Autodesk Fusion 360 part; units mm, degrees
note: some values were not read from the file. Chosen so that the rebuilt part matches the saved one: which bodies a step acts on; which pieces of a blend or face edit are solid. Set by a fixed rule: which sketch regions a step uses.
(part 3 of 4)
  spline S7 degree 5 poles (-3.4009, 1.0262) (-3.3954, 1.0308) (-3.3845, 1.0401) (-3.3681, 1.0541) (-3.3463, 1.0727) (-3.3193, 1.0962) (-3.2925, 1.1198) (-3.2658, 1.1434) (-3.2393, 1.1672) (-3.213, 1.191) (-3.1868, 1.215) (-3.1608, 1.239) (-3.135, 1.2632) (-3.1094, 1.2874) (-3.084, 1.3118) (-3.0587, 1.3362) (-3.0337, 1.3607) (-3.0088, 1.3854) (-2.9841, 1.4101) (-2.9595, 1.4349) (-2.9352, 1.4598) (-2.9111, 1.4848) (-2.8871, 1.5099) (-2.8634, 1.5352) (-2.8398, 1.5604) (-2.8165, 1.5858) (-2.7933, 1.6113) (-2.7703, 1.6369) (-2.7476, 1.6626) (-2.725, 1.6883) (-2.7027, 1.7142) (-2.6805, 1.7401) (-2.6586, 1.7662) (-2.6369, 1.7923) (-2.6154, 1.8185) (-2.5941, 1.8448) (-2.5731, 1.8713) (-2.5522, 1.8977) (-2.5316, 1.9243) (-2.5112, 1.951) (-2.491, 1.9778) (-2.4711, 2.0047) (-2.4514, 2.0316) (-2.432, 2.0587) (-2.4128, 2.0858) (-2.3939, 2.113) (-2.3751, 2.1403) (-2.3567, 2.1678) (-2.3385, 2.1953) (-2.3205, 2.2228) (-2.3029, 2.2505) (-2.2855, 2.2783) (-2.2684, 2.3062) (-2.2516, 2.3342) (-2.2352, 2.3622) (-2.219, 2.3904) (-2.203, 2.4187) (-2.1874, 2.447) (-2.172, 2.4754) (-2.157, 2.5039) (-2.1423, 2.5326) (-2.1281, 2.5613) (-2.1144, 2.5902) (-2.1011, 2.6192) (-2.0883, 2.6484) (-2.0758, 2.6776) (-2.0636, 2.7069) (-2.0515, 2.7362) (-2.0398, 2.7656) (-2.0288, 2.7952) (-2.0187, 2.825) (-2.0118, 2.8491) (-2.0073, 2.8674) (-2.0047, 2.8797) (-2.0035, 2.8858) knots -1 -1 -1 -1 -1 -1 -0.98571429 -0.97142857 -0.95714286 -0.94285714 -0.92857143 -0.91428571 -0.9 -0.88571429 -0.87142857 -0.85714286 -0.84285714 -0.82857143 -0.81428571 -0.8 -0.78571429 -0.77142857 -0.75714286 -0.74285714 -0.72857143 -0.71428571 -0.7 -0.68571429 -0.67142857 -0.65714286 -0.64285714 -0.62857143 -0.61428571 -0.6 -0.58571429 -0.57142857 -0.55714286 -0.54285714 -0.52857143 -0.51428571 -0.5 -0.48571429 -0.47142857 -0.45714286 -0.44285714 -0.42857143 -0.41428571 -0.4 -0.38571429 -0.37142857 -0.35714286 -0.34285714 -0.32857143 -0.31428571 -0.3 -0.28571429 -0.27142857 -0.25714286 -0.24285714 -0.22857143 -0.21428571 -0.2 -0.18571429 -0.17142857 -0.15714286 -0.14285714 -0.12857143 -0.11428571 -0.1 -0.08571429 -0.07142857 -0.05714286 -0.04285714 -0.02857143 -0.01428571 0 0 0 0 0 0
  line L7 (-2.0035, 2.8858) -> (-1.9517, 3.1488)
  arc A15 (-1.0746, 3.7888) -> (-1.9517, 3.1488) centre (-1.1668, 2.9941) ccw
  arc A16 (-1.0746, 3.7888) -> (-0.8753, 3.7678) centre (0, 13.0546) ccw
  arc A17 (-0.1505, 2.9594) -> (-0.8753, 3.7678) centre (-0.9504, 2.9714) ccw
  line L8 (-0.1505, 2.9594) -> (-0.1545, 2.6915)
  spline S8 degree 5 poles (-0.1545, 2.6915) (-0.1546, 2.6852) (-0.1546, 2.6727) (-0.154, 2.6538) (-0.1523, 2.6288) (-0.1486, 2.5976) (-0.1439, 2.5664) (-0.1386, 2.5352) (-0.133, 2.504) (-0.127, 2.4728) (-0.1209, 2.4416) (-0.1144, 2.4104) (-0.1075, 2.3793) (-0.1001, 2.3482) (-0.0922, 2.3171) (-0.0838, 2.286) (-0.075, 2.255) (-0.0659, 2.224) (-0.0564, 2.193) (-0.0467, 2.1621) (-0.0368, 2.1312) (-0.0265, 2.1003) (-0.0159, 2.0694) (-0.005, 2.0386) (0.0062, 2.0078) (0.0178, 1.9771) (0.0296, 1.9464) (0.0417, 1.9157) (0.054, 1.885) (0.0667, 1.8544) (0.0795, 1.8238) (0.0927, 1.7933) (0.1061, 1.7628) (0.1197, 1.7323) (0.1336, 1.7019) (0.1478, 1.6716) (0.1622, 1.6412) (0.1768, 1.6109) (0.1917, 1.5807) (0.2068, 1.5505) (0.2221, 1.5203) (0.2377, 1.4902) (0.2535, 1.4601) (0.2695, 1.4301) (0.2858, 1.4001) (0.3023, 1.3701) (0.319, 1.3403) (0.3359, 1.3104) (0.3531, 1.2806) (0.3704, 1.2509) (0.388, 1.2212) (0.4058, 1.1916) (0.4238, 1.162) (0.442, 1.1324) (0.4604, 1.1029) (0.479, 1.0735) (0.4978, 1.0441) (0.5168, 1.0148) (0.5361, 0.9855) (0.5555, 0.9563) (0.5751, 0.9272) (0.5949, 0.8981) (0.615, 0.869) (0.6352, 0.84) (0.6556, 0.8111) (0.6762, 0.7823) (0.697, 0.7534) (0.718, 0.7247) (0.7391, 0.696) (0.7605, 0.6674) (0.782, 0.6388) (0.7994, 0.616) (0.8126, 0.599) (0.8214, 0.5876) (0.8258, 0.5819) knots 0 0 0 0 0 0 0.01428571 0.02857143 0.04285714 0.05714286 0.07142857 0.08571429 0.1 0.11428571 0.12857143 0.14285714 0.15714286 0.17142857 0.18571429 0.2 0.21428571 0.22857143 0.24285714 0.25714286 0.27142857 0.28571429 0.3 0.31428571 0.32857143 0.34285714 0.35714286 0.37142857 0.38571429 0.4 0.41428571 0.42857143 0.44285714 0.45714286 0.47142857 0.48571429 0.5 0.51428571 0.52857143 0.54285714 0.55714286 0.57142857 0.58571429 0.6 0.61428571 0.62857143 0.64285714 0.65714286 0.67142857 0.68571429 0.7 0.71428571 0.72857143 0.74285714 0.75714286 0.77142857 0.78571429 0.8 0.81428571 0.82857143 0.84285714 0.85714286 0.87142857 0.88571429 0.9 0.91428571 0.92857143 0.94285714 0.95714286 0.97142857 0.98571429 1 1 1 1 1 1
  arc A18 (0.8258, 0.5819) -> (1.7855, 0.6828) centre (0, 13.0546) ccw
  spline S9 degree 5 poles (1.7855, 0.6828) (1.7886, 0.6893) (1.7949, 0.7022) (1.8042, 0.7216) (1.8164, 0.7476) (1.8316, 0.78) (1.8465, 0.8124) (1.8613, 0.8449) (1.8758, 0.8773) (1.8902, 0.9098) (1.9043, 0.9424) (1.9183, 0.9749) (1.932, 1.0075) (1.9455, 1.04) (1.9589, 1.0726) (1.972, 1.1052) (1.985, 1.1378) (1.9977, 1.1704) (2.0102, 1.2031) (2.0225, 1.2357) (2.0346, 1.2684) (2.0465, 1.3011) (2.0581, 1.3337) (2.0696, 1.3664) (2.0808, 1.3991) (2.0918, 1.4318) (2.1026, 1.4645) (2.1132, 1.4972) (2.1235, 1.5299) (2.1336, 1.5626) (2.1435, 1.5953) (2.1532, 1.628) (2.1627, 1.6608) (2.1719, 1.6935) (2.1808, 1.7262) (2.1896, 1.7589) (2.1981, 1.7915) (2.2063, 1.8242) (2.2144, 1.8569) (2.2221, 1.8896) (2.2297, 1.9222) (2.2369, 1.9549) (2.244, 1.9875) (2.2507, 2.0201) (2.2572, 2.0527) (2.2634, 2.0853) (2.2694, 2.1179) (2.2751, 2.1504) (2.2806, 2.1829) (2.2858, 2.2155) (2.2906, 2.2479) (2.2952, 2.2804) (2.2995, 2.3128) (2.3034, 2.3452) (2.3071, 2.3775) (2.3104, 2.4098) (2.3135, 2.4421) (2.3162, 2.4744) (2.3187, 2.5066) (2.3209, 2.5388) (2.3226, 2.5709) (2.3239, 2.6029) (2.3247, 2.6349) (2.325, 2.6668) (2.3248, 2.6987) (2.3244, 2.7304) (2.3236, 2.7622) (2.3227, 2.7939) (2.3214, 2.8255) (2.3195, 2.857) (2.3166, 2.8883) (2.3131, 2.9132) (2.3097, 2.9317) (2.3071, 2.944) (2.3057, 2.9501) knots -1 -1 -1 -1 -1 -1 -0.98571429 -0.97142857 -0.95714286 -0.94285714 -0.92857143 -0.91428571 -0.9 -0.88571429 -0.87142857 -0.85714286 -0.84285714 -0.82857143 -0.81428571 -0.8 -0.78571429 -0.77142857 -0.75714286 -0.74285714 -0.72857143 -0.71428571 -0.7 -0.68571429 -0.67142857 -0.65714286 -0.64285714 -0.62857143 -0.61428571 -0.6 -0.58571429 -0.57142857 -0.55714286 -0.54285714 -0.52857143 -0.51428571 -0.5 -0.48571429 -0.47142857 -0.45714286 -0.44285714 -0.42857143 -0.41428571 -0.4 -0.38571429 -0.37142857 -0.35714286 -0.34285714 -0.32857143 -0.31428571 -0.3 -0.28571429 -0.27142857 -0.25714286 -0.24285714 -0.22857143 -0.21428571 -0.2 -0.18571429 -0.17142857 -0.15714286 -0.14285714 -0.12857143 -0.11428571 -0.1 -0.08571429 -0.07142857 -0.05714286 -0.04285714 -0.02857143 -0.01428571 0 0 0 0 0 0
  line L9 (2.3057, 2.9501) -> (2.2461, 3.2113)
  arc A19 (2.787, 4.1528) -> (2.2461, 3.2113) centre (3.026, 3.3893) ccw
  arc A20 (2.787, 4.1528) -> (2.9776, 4.2147) centre (0, 13.0546) ccw
  arc A21 (3.9686, 3.771) -> (2.9776, 4.2147) centre (3.233, 3.4565) ccw
  line L10 (3.9686, 3.771) -> (4.0739, 3.5246)
  spline S10 degree 5 poles (4.0739, 3.5246) (4.0764, 3.5188) (4.0815, 3.5074) (4.0897, 3.4904) (4.1015, 3.4682) (4.1175, 3.4412) (4.1345, 3.4146) (4.152, 3.3882) (4.1699, 3.3621) (4.188, 3.336) (4.2063, 3.31) (4.2249, 3.2841) (4.2438, 3.2585) (4.2633, 3.2331) (4.2831, 3.2079) (4.3034, 3.1829) (4.3241, 3.1582) (4.345, 3.1336) (4.3662, 3.1091) (4.3877, 3.0848) (4.4094, 3.0606) (4.4313, 3.0366) (4.4536, 3.0127) (4.4761, 2.989) (4.4988, 2.9654) (4.5219, 2.942) (4.5452, 2.9188) (4.5687, 2.8956) (4.5924, 2.8727) (4.6164, 2.8498) (4.6406, 2.8271) (4.665, 2.8046) (4.6897, 2.7822) (4.7145, 2.7599) (4.7396, 2.7378) (4.7649, 2.7158) (4.7904, 2.6939) (4.8161, 2.6722) (4.842, 2.6506) (4.8681, 2.6292) (4.8944, 2.6078) (4.9208, 2.5867) (4.9475, 2.5656) (4.9744, 2.5447) (5.0014, 2.5239) (5.0287, 2.5033) (5.0561, 2.4828) (5.0837, 2.4624) (5.1115, 2.4421) (5.1394, 2.422) (5.1675, 2.4021) (5.1958, 2.3822) (5.2243, 2.3625) (5.2529, 2.3429) (5.2818, 2.3235) (5.3107, 2.3042) (5.3399, 2.285) (5.3692, 2.2659) (5.3987, 2.247) (5.4283, 2.2282) (5.4581, 2.2096) (5.488, 2.191) (5.5181, 2.1727) (5.5484, 2.1544) (5.5788, 2.1363) (5.6093, 2.1183) (5.6401, 2.1004) (5.6709, 2.0827) (5.7019, 2.0651) (5.7331, 2.0476) (5.7644, 2.0303) (5.7895, 2.0166) (5.8085, 2.0063) (5.8211, 1.9995) (5.8275, 1.9961) knots 0 0 0 0 0 0 0.01428571 0.02857143 0.04285714 0.05714286 0.07142857 0.08571429 0.1 0.11428571 0.12857143 0.14285714 0.15714286 0.17142857 0.18571429 0.2 0.21428571 0.22857143 0.24285714 0.25714286 0.27142857 0.28571429 0.3 0.31428571 0.32857143 0.34285714 0.35714286 0.37142857 0.38571429 0.4 0.41428571 0.42857143 0.44285714 0.45714286 0.47142857 0.48571429 0.5 0.51428571 0.52857143 0.54285714 0.55714286 0.57142857 0.58571429 0.6 0.61428571 0.62857143 0.64285714 0.65714286 0.67142857 0.68571429 0.7 0.71428571 0.72857143 0.74285714 0.75714286 0.77142857 0.78571429 0.8 0.81428571 0.82857143 0.84285714 0.85714286 0.87142857 0.88571429 0.9 0.91428571 0.92857143 0.94285714 0.95714286 0.97142857 0.98571429 1 1 1 1 1 1
  arc A22 (5.8275, 1.9961) -> (6.6632, 2.4786) centre (0, 13.0546) ccw
  spline S11 degree 5 poles (6.6632, 2.4786) (6.6634, 2.4858) (6.6639, 2.5002) (6.6645, 2.5217) (6.6651, 2.5504) (6.6658, 2.5861) (6.6662, 2.6218) (6.6665, 2.6575) (6.6666, 2.6931) (6.6665, 2.7286) (6.6662, 2.7641) (6.6657, 2.7995) (6.665, 2.8348) (6.6641, 2.8701) (6.6631, 2.9053) (6.6618, 2.9404) (6.6603, 2.9754) (6.6587, 3.0104) (6.6568, 3.0453) (6.6548, 3.0801) (6.6526, 3.1149) (6.6501, 3.1496) (6.6475, 3.1842) (6.6447, 3.2187) (6.6416, 3.2531) (6.6384, 3.2875) (6.6349, 3.3217) (6.6313, 3.3559) (6.6274, 3.39) (6.6234, 3.424) (6.6191, 3.4579) (6.6147, 3.4917) (6.61, 3.5254) (6.6051, 3.5591) (6.6, 3.5926) (6.5947, 3.626) (6.5891, 3.6593) (6.5834, 3.6926) (6.5774, 3.7257) (6.5713, 3.7587) (6.5649, 3.7916) (6.5582, 3.8243) (6.5514, 3.857) (6.5443, 3.8896) (6.5369, 3.922) (6.5294, 3.9543) (6.5216, 3.9865) (6.5136, 4.0185) (6.5053, 4.0505) (6.4968, 4.0822) (6.4881, 4.1139) (6.4791, 4.1454) (6.4698, 4.1768) (6.4602, 4.2079) (6.4504, 4.239) (6.4403, 4.2699) (6.4299, 4.3006) (6.4194, 4.3312) (6.4085, 4.3616) (6.3974, 4.3919) (6.3859, 4.4219) (6.3741, 4.4517) (6.3618, 4.4813) (6.3491, 4.5105) (6.336, 4.5396) (6.3226, 4.5684) (6.3091, 4.5971) (6.2953, 4.6257) (6.2813, 4.654) (6.2667, 4.682) (6.2513, 4.7095) (6.238, 4.7307) (6.2274, 4.7463) (6.22, 4.7564) (6.2162, 4.7615) knots -1 -1 -1 -1 -1 -1 -0.98571429 -0.97142857 -0.95714286 -0.94285714 -0.92857143 -0.91428571 -0.9 -0.88571429 -0.87142857 -0.85714286 -0.84285714 -0.82857143 -0.81428571 -0.8 -0.78571429 -0.77142857 -0.75714286 -0.74285714 -0.72857143 -0.71428571 -0.7 -0.68571429 -0.67142857 -0.65714286 -0.64285714 -0.62857143 -0.61428571 -0.6 -0.58571429 -0.57142857 -0.55714286 -0.54285714 -0.52857143 -0.51428571 -0.5 -0.48571429 -0.47142857 -0.45714286 -0.44285714 -0.42857143 -0.41428571 -0.4 -0.38571429 -0.37142857 -0.35714286 -0.34285714 -0.32857143 -0.31428571 -0.3 -0.28571429 -0.27142857 -0.25714286 -0.24285714 -0.22857143 -0.21428571 -0.2 -0.18571429 -0.17142857 -0.15714286 -0.14285714 -0.12857143 -0.11428571 -0.1 -0.08571429 -0.07142857 -0.05714286 -0.04285714 -0.02857143 -0.01428571 0 0 0 0 0 0
  line L11 (6.2162, 4.7615) -> (6.0555, 4.9759)
  arc A23 (6.1668, 6.0559) -> (6.0555, 4.9759) centre (6.6957, 5.4557) ccw
  arc A24 (6.1668, 6.0559) -> (6.3157, 6.1901) centre (0, 13.0546) ccw
  arc A25 (7.4015, 6.1878) -> (6.3157, 6.1901) centre (6.8574, 5.6013) ccw
  line L12 (7.4015, 6.1878) -> (7.5979, 6.0055)
  spline S12 degree 5 poles (7.5979, 6.0055) (7.6025, 6.0013) (7.6119, 5.9929) (7.6262, 5.9807) (7.646, 5.9652) (7.6717, 5.947) (7.698, 5.9296) (7.7247, 5.9127) (7.7517, 5.8961) (7.7788, 5.8796) (7.8061, 5.8633) (7.8336, 5.8472) (7.8614, 5.8315) (7.8895, 5.8162) (7.9179, 5.8013) (7.9465, 5.7867) (7.9755, 5.7725) (8.0046, 5.7586) (8.034, 5.7449) (8.0634, 5.7314) (8.0931, 5.7181) (8.1229, 5.7051) (8.1529, 5.6923) (8.1831, 5.6798) (8.2135, 5.6675) (8.2441, 5.6555) (8.2748, 5.6437) (8.3057, 5.6322) (8.3368, 5.6209) (8.368, 5.6098) (8.3993, 5.5989) (8.4308, 5.5882) (8.4624, 5.5777) (8.4942, 5.5675) (8.5261, 5.5575) (8.5581, 5.5477) (8.5903, 5.5381) (8.6226, 5.5287) (8.6551, 5.5195) (8.6876, 5.5105) (8.7203, 5.5017) (8.7531, 5.4931) (8.786, 5.4848) (8.8191, 5.4766) (8.8522, 5.4686) (8.8855, 5.4608) (8.9189, 5.4532) (8.9524, 5.4458) (8.986, 5.4387) (9.0197, 5.4317) (9.0536, 5.4248) (9.0875, 5.4182) (9.1215, 5.4118) (9.1556, 5.4056) (9.1899, 5.3995) (9.2242, 5.3936) (9.2586, 5.388) (9.2931, 5.3825) (9.3278, 5.3772) (9.3625, 5.3721) (9.3973, 5.3672) (9.4322, 5.3624) (9.4671, 5.3579) (9.5022, 5.3535) (9.5374, 5.3493) (9.5726, 5.3453) (9.6079, 5.3415) (9.6433, 5.3378) (9.6788, 5.3344) (9.7144, 5.3311) (9.75, 5.328) (9.7786, 5.3257) (9.8001, 5.324) (9.8144, 5.3229) (9.8216, 5.3224) knots 0 0 0 0 0 0 0.01428571 0.02857143 0.04285714 0.05714286 0.07142857 0.08571429 0.1 0.11428571 0.12857143 0.14285714 0.15714286 0.17142857 0.18571429 0.2 0.21428571 0.22857143 0.24285714 0.25714286 0.27142857 0.28571429 0.3 0.31428571 0.32857143 0.34285714 0.35714286 0.37142857 0.38571429 0.4 0.41428571 0.42857143 0.44285714 0.45714286 0.47142857 0.48571429 0.5 0.51428571 0.52857143 0.54285714 0.55714286 0.57142857 0.58571429 0.6 0.61428571 0.62857143 0.64285714 0.65714286 0.67142857 0.68571429 0.7 0.71428571 0.72857143 0.74285714 0.75714286 0.77142857 0.78571429 0.8 0.81428571 0.82857143 0.84285714 0.85714286 0.87142857 0.88571429 0.9 0.91428571 0.92857143 0.94285714 0.95714286 0.97142857 0.98571429 1 1 1 1 1 1
  arc A26 (9.8216, 5.3224) -> (10.3888, 6.1031) centre (0, 13.0546) ccw
  spline S13 degree 5 poles (10.3888, 6.1031) (10.3861, 6.1098) (10.3806, 6.1231) (10.3724, 6.143) (10.3614, 6.1694) (10.3474, 6.2024) (10.3333, 6.2352) (10.319, 6.2679) (10.3046, 6.3004) (10.2901, 6.3328) (10.2754, 6.3651) (10.2605, 6.3973) (10.2455, 6.4292) (10.2304, 6.4611) (10.2151, 6.4928) (10.1997, 6.5244) (10.1841, 6.5558) (10.1684, 6.5871) (10.1525, 6.6182) (10.1364, 6.6492) (10.1203, 6.6801) (10.1039, 6.7108) (10.0875, 6.7413) (10.0708, 6.7717) (10.054, 6.8019) (10.0371, 6.832) (10.02, 6.8619) (10.0028, 6.8916) (9.9854, 6.9212) (9.9679, 6.9506) (9.9502, 6.9798) (9.9324, 7.0089) (9.9144, 7.0378) (9.8962, 7.0665) (9.8779, 7.0951) (9.8595, 7.1235) (9.8409, 7.1516) (9.8221, 7.1797) (9.8032, 7.2075) (9.7841, 7.2351) (9.7649, 7.2626) (9.7455, 7.2898) (9.726, 7.3169) (9.7062, 7.3437) (9.6864, 7.3703) (9.6663, 7.3968) (9.6461, 7.423) (9.6258, 7.449) (9.6052, 7.4749) (9.5845, 7.5004) (9.5637, 7.5258) (9.5426, 7.5509) (9.5214, 7.5758) (9.5, 7.6004) (9.4783, 7.6247) (9.4566, 7.6488) (9.4346, 7.6727) (9.4125, 7.6964) (9.3902, 7.7198) (9.3678, 7.7429) (9.3451, 7.7657) (9.3221, 7.7881) (9.2989, 7.81) (9.2753, 7.8316) (9.2516, 7.8528) (9.2276, 7.8737) (9.2036, 7.8944) (9.1794, 7.9149) (9.1551, 7.9351) (9.1304, 7.9548) (9.1051, 7.9736) (9.0843, 7.9876) (9.0683, 7.9975) (9.0574, 8.0038) (9.0519, 8.0068) knots -1 -1 -1 -1 -1 -1 -0.98571429 -0.97142857 -0.95714286 -0.94285714 -0.92857143 -0.91428571 -0.9 -0.88571429 -0.87142857 -0.85714286 -0.84285714 -0.82857143 -0.81428571 -0.8 -0.78571429 -0.77142857 -0.75714286 -0.74285714 -0.72857143 -0.71428571 -0.7 -0.68571429 -0.67142857 -0.65714286 -0.64285714 -0.62857143 -0.61428571 -0.6 -0.58571429 -0.57142857 -0.55714286 -0.54285714 -0.52857143 -0.51428571 -0.5 -0.48571429 -0.47142857 -0.45714286 -0.44285714 -0.42857143 -0.41428571 -0.4 -0.38571429 -0.37142857 -0.35714286 -0.34285714 -0.32857143 -0.31428571 -0.3 -0.28571429 -0.27142857 -0.25714286 -0.24285714 -0.22857143 -0.21428571 -0.2 -0.18571429 -0.17142857 -0.15714286 -0.14285714 -0.12857143 -0.11428571 -0.1 -0.08571429 -0.07142857 -0.05714286 -0.04285714 -0.02857143 -0.01428571 0 0 0 0 0 0
  line L13 (9.0519, 8.0068) -> (8.8179, 8.1373)
  arc A27 (8.4802, 9.1693) -> (8.8179, 8.1373) centre (9.2075, 8.836) ccw
  arc A28 (8.4802, 9.1693) -> (8.5618, 9.3524) centre (0, 13.0546) ccw
  arc A29 (9.5546, 9.7919) -> (8.5618, 9.3524) centre (9.2961, 9.0348) ccw
  line L14 (9.5546, 9.7919) -> (9.8082, 9.7053)
  spline S14 degree 5 poles (9.8082, 9.7053) (9.8141, 9.7033) (9.8261, 9.6994) (9.8441, 9.6941) (9.8685, 9.6881) (9.8993, 9.6819) (9.9304, 9.6767) (9.9617, 9.6721) (9.9932, 9.6678) (10.0246, 9.6638) (10.0562, 9.66) (10.0879, 9.6566) (10.1196, 9.6535) (10.1515, 9.6509) (10.1835, 9.6489) (10.2156, 9.6472) (10.2479, 9.646) (10.2802, 9.6451) (10.3125, 9.6445) (10.345, 9.6442) (10.3774, 9.6441) (10.41, 9.6444) (10.4426, 9.6449) (10.4753, 9.6457) (10.508, 9.6469) (10.5409, 9.6484) (10.5737, 9.6501) (10.6066, 9.6521) (10.6396, 9.6544) (10.6726, 9.657) (10.7057, 9.6598) (10.7388, 9.6628) (10.7719, 9.6661) (10.8051, 9.6697) (10.8383, 9.6735) (10.8716, 9.6776) (10.9049, 9.6819) (10.9382, 9.6865) (10.9716, 9.6913) (11.005, 9.6963) (11.0384, 9.7016) (11.0719, 9.7071) (11.1054, 9.7128) (11.1389, 9.7188) (11.1724, 9.725) (11.206, 9.7314) (11.2396, 9.7381) (11.2732, 9.7449) (11.3068, 9.752) (11.3405, 9.7593) (11.3741, 9.7669) (11.4078, 9.7746) (11.4415, 9.7826) (11.4752, 9.7908) (11.509, 9.7992) (11.5427, 9.8078) (11.5765, 9.8166) (11.6102, 9.8256) (11.644, 9.8349) (11.6778, 9.8443) (11.7116, 9.854) (11.7454, 9.8639) (11.7792, 9.8739) (11.813, 9.8842) (11.8468, 9.8947) (11.8807, 9.9053) (11.9145, 9.9162) (11.9483, 9.9273) (11.9821, 9.9386) (12.0159, 9.95) (12.0498, 9.9617) (12.0768, 9.9712) (12.0971, 9.9784) (12.1106, 9.9832) (12.1174, 9.9857) knots 0 0 0 0 0 0 0.01428571 0.02857143 0.04285714 0.05714286 0.07142857 0.08571429 0.1 0.11428571 0.12857143 0.14285714 0.15714286 0.17142857 0.18571429 0.2 0.21428571 0.22857143 0.24285714 0.25714286 0.27142857 0.28571429 0.3 0.31428571 0.32857143 0.34285714 0.35714286 0.37142857 0.38571429 0.4 0.41428571 0.42857143 0.44285714 0.45714286 0.47142857 0.48571429 0.5 0.51428571 0.52857143 0.54285714 0.55714286 0.57142857 0.58571429 0.6 0.61428571 0.62857143 0.64285714 0.65714286 0.67142857 0.68571429 0.7 0.71428571 0.72857143 0.74285714 0.75714286 0.77142857 0.78571429 0.8 0.81428571 0.82857143 0.84285714 0.85714286 0.87142857 0.88571429 0.9 0.91428571 0.92857143 0.94285714 0.95714286 0.97142857 0.98571429 1 1 1 1 1 1
  arc A30 (12.1174, 9.9857) -> (12.3181, 10.9296) centre (0, 13.0546) ccw
  spline S15 degree 5 poles (12.3181, 10.9296) (12.3129, 10.9346) (12.3025, 10.9445) (12.2869, 10.9594) (12.266, 10.979) (12.2399, 11.0035) (12.2136, 11.0277) (12.1873, 11.0518) (12.1609, 11.0756) (12.1344, 11.0993) (12.1079, 11.1228) (12.0813, 11.1461) (12.0545, 11.1693) (12.0278, 11.1922) (12.0009, 11.215) (11.9739, 11.2375) (11.9469, 11.2599) (11.9198, 11.2821) (11.8926, 11.3041) (11.8654, 11.3259) (11.8381, 11.3475) (11.8107, 11.3689) (11.7832, 11.39) (11.7557, 11.411) (11.728, 11.4318) (11.7003, 11.4524) (11.6726, 11.4728) (11.6447, 11.4929) (11.6168, 11.5129) (11.5889, 11.5326) (11.5608, 11.5521) (11.5327, 11.5714) (11.5045, 11.5905) (11.4762, 11.6094) (11.4479, 11.628) (11.4195, 11.6464) (11.3911, 11.6646) (11.3625, 11.6826) (11.3339, 11.7003) (11.3053, 11.7178) (11.2765, 11.7351) (11.2477, 11.7521) (11.2189, 11.7688) (11.1899, 11.7853) (11.1609, 11.8016) (11.1319, 11.8176) (11.1027, 11.8333) (11.0736, 11.8488) (11.0443, 11.8641) (11.015, 11.879) (10.9856, 11.8937) (10.9562, 11.9081) (10.9267, 11.9221) (10.8971, 11.9359) (10.8674, 11.9494) (10.8377, 11.9625) (10.808, 11.9754) (10.7782, 11.988) (10.7483, 12.0003) (10.7184, 12.0123) (10.6883, 12.0239) (10.6583, 12.035) (10.6281, 12.0457) (10.5978, 12.0558) (10.5675, 12.0655) (10.5371, 12.0749) (10.5067, 12.084) (10.4763, 12.0929) (10.4458, 12.1014) (10.4153, 12.1093) (10.3846, 12.1162) (10.3599, 12.1206) (10.3412, 12.1231) (10.3287, 12.1244) (10.3225, 12.125) knots -1 -1 -1 -1 -1 -1 -0.98571429 -0.97142857 -0.95714286 -0.94285714 -0.92857143 -0.91428571 -0.9 -0.88571429 -0.87142857 -0.85714286 -0.84285714 -0.82857143 -0.81428571 -0.8 -0.78571429 -0.77142857 -0.75714286 -0.74285714 -0.72857143 -0.71428571 -0.7 -0.68571429 -0.67142857 -0.65714286 -0.64285714 -0.62857143 -0.61428571 -0.6 -0.58571429 -0.57142857 -0.55714286 -0.54285714 -0.52857143 -0.51428571 -0.5 -0.48571429 -0.47142857 -0.45714286 -0.44285714 -0.42857143 -0.41428571 -0.4 -0.38571429 -0.37142857 -0.35714286 -0.34285714 -0.32857143 -0.31428571 -0.3 -0.28571429 -0.27142857 -0.25714286 -0.24285714 -0.22857143 -0.21428571 -0.2 -0.18571429 -0.17142857 -0.15714286 -0.14285714 -0.12857143 -0.11428571 -0.1 -0.08571429 -0.07142857 -0.05714286 -0.04285714 -0.02857143 -0.01428571 0 0 0 0 0 0
  line L15 (10.3225, 12.125) -> (10.0556, 12.149)
  arc A31 (9.3274, 12.9544) -> (10.0556, 12.149) centre (10.1274, 12.9458) ccw
  arc A32 (9.3274, 12.9544) -> (9.3274, 13.1548) centre (0, 13.0546) ccw
  arc A33 (10.0556, 13.9602) -> (9.3274, 13.1548) centre (10.1274, 13.1634) ccw
  line L16 (10.0556, 13.9602) -> (10.3225, 13.9842)
  spline S16 degree 5 poles (10.3225, 13.9842) (10.3287, 13.9848) (10.3412, 13.9861) (10.3599, 13.9886) (10.3846, 13.993) (10.4153, 13.9999) (10.4458, 14.0078) (10.4763, 14.0163) (10.5067, 14.0252) (10.5371, 14.0344) (10.5675, 14.0437) (10.5978, 14.0534) (10.6281, 14.0636) (10.6583, 14.0742) (10.6883, 14.0853) (10.7184, 14.0969) (10.7483, 14.1089) (10.7782, 14.1212) (10.808, 14.1338) (10.8377, 14.1467) (10.8674, 14.1599) (10.8971, 14.1733) (10.9267, 14.1871) (10.9562, 14.2011) (10.9856, 14.2155) (11.015, 14.2302) (11.0443, 14.2452) (11.0736, 14.2604) (11.1027, 14.2759) (11.1319, 14.2916) (11.1609, 14.3076) (11.1899, 14.3239) (11.2189, 14.3404) (11.2477, 14.3572) (11.2765, 14.3742) (11.3053, 14.3914) (11.3339, 14.4089) (11.3625, 14.4266) (11.3911, 14.4446) (11.4195, 14.4628) (11.4479, 14.4812) (11.4762, 14.4998) (11.5045, 14.5187) (11.5327, 14.5378) (11.5608, 14.5571) (11.5889, 14.5766) (11.6168, 14.5963) (11.6447, 14.6163) (11.6726, 14.6365) (11.7003, 14.6568) (11.728, 14.6774) (11.7557, 14.6982) (11.7832, 14.7192) (11.8107, 14.7404) (11.8381, 14.7618) (11.8654, 14.7833) (11.8926, 14.8051) (11.9198, 14.8271) (11.9469, 14.8493) (11.9739, 14.8717) (12.0009, 14.8942) (12.0278, 14.917) (12.0545, 14.9399) (12.0813, 14.9631) (12.1079, 14.9864) (12.1344, 15.0099) (12.1609, 15.0336) (12.1873, 15.0575) (12.2136, 15.0815) (12.2399, 15.1058) (12.266, 15.1302) (12.2869, 15.1499) (12.3025, 15.1647) (12.3129, 15.1746) (12.3181, 15.1796) knots 0 0 0 0 0 0 0.01428571 0.02857143 0.04285714 0.05714286 0.07142857 0.08571429 0.1 0.11428571 0.12857143 0.14285714 0.15714286 0.17142857 0.18571429 0.2 0.21428571 0.22857143 0.24285714 0.25714286 0.27142857 0.28571429 0.3 0.31428571 0.32857143 0.34285714 0.35714286 0.37142857 0.38571429 0.4 0.41428571 0.42857143 0.44285714 0.45714286 0.47142857 0.48571429 0.5 0.51428571 0.52857143 0.54285714 0.55714286 0.57142857 0.58571429 0.6 0.61428571 0.62857143 0.64285714 0.65714286 0.67142857 0.68571429 0.7 0.71428571 0.72857143 0.74285714 0.75714286 0.77142857 0.78571429 0.8 0.81428571 0.82857143 0.84285714 0.85714286 0.87142857 0.88571429 0.9 0.91428571 0.92857143 0.94285714 0.95714286 0.97142857 0.98571429 1 1 1 1 1 1
  arc A34 (12.3181, 15.1796) -> (12.1174, 16.1235) centre (0, 13.0546) ccw
  spline S17 degree 5 poles (12.1174, 16.1235) (12.1106, 16.126) (12.0971, 16.1308) (12.0768, 16.138) (12.0498, 16.1475) (12.0159, 16.1592) (11.9821, 16.1707) (11.9483, 16.1819) (11.9145, 16.193) (11.8807, 16.2039) (11.8468, 16.2146) (11.813, 16.225) (11.7792, 16.2353) (11.7454, 16.2454) (11.7116, 16.2552) (11.6778, 16.2649) (11.644, 16.2743) (11.6102, 16.2836) (11.5765, 16.2926) (11.5427, 16.3014) (11.509, 16.31) (11.4752, 16.3184) (11.4415, 16.3266) (11.4078, 16.3346) (11.3741, 16.3423) (11.3405, 16.3499) (11.3068, 16.3572) (11.2732, 16.3643) (11.2396, 16.3712) (11.206, 16.3778) (11.1724, 16.3842) (11.1389, 16.3904) (11.1054, 16.3964) (11.0719, 16.4021) (11.0384, 16.4076) (11.005, 16.4129) (10.9716, 16.418) (10.9382, 16.4228) (10.9049, 16.4273) (10.8716, 16.4316) (10.8383, 16.4357) (10.8051, 16.4395) (10.7719, 16.4431) (10.7388, 16.4464) (10.7057, 16.4495) (10.6726, 16.4523) (10.6396, 16.4548) (10.6066, 16.4571) (10.5737, 16.4591) (10.5409, 16.4608) (10.508, 16.4623) (10.4753, 16.4635) (10.4426, 16.4643) (10.41, 16.4649) (10.3774, 16.4651) (10.345, 16.465) (10.3125, 16.4647) (10.2802, 16.4641) (10.2479, 16.4632) (10.2156, 16.462) (10.1835, 16.4604) (10.1515, 16.4583) (10.1196, 16.4557) (10.0879, 16.4527) (10.0562, 16.4492) (10.0246, 16.4454) (9.9932, 16.4414) (9.9617, 16.4371) (9.9304, 16.4325) (9.8993, 16.4274) (9.8685, 16.4212) (9.8441, 16.4151) (9.8261, 16.4098) (9.8141, 16.4059) (9.8082, 16.4039) knots -1 -1 -1 -1 -1 -1 -0.98571429 -0.97142857 -0.95714286 -0.94285714 -0.92857143 -0.91428571 -0.9 -0.88571429 -0.87142857 -0.85714286 -0.84285714 -0.82857143 -0.81428571 -0.8 -0.78571429 -0.77142857 -0.75714286 -0.74285714 -0.72857143 -0.71428571 -0.7 -0.68571429 -0.67142857 -0.65714286 -0.64285714 -0.62857143 -0.61428571 -0.6 -0.58571429 -0.57142857 -0.55714286 -0.54285714 -0.52857143 -0.51428571 -0.5 -0.48571429 -0.47142857 -0.45714286 -0.44285714 -0.42857143 -0.41428571 -0.4 -0.38571429 -0.37142857 -0.35714286 -0.34285714 -0.32857143 -0.31428571 -0.3 -0.28571429 -0.27142857 -0.25714286 -0.24285714 -0.22857143 -0.21428571 -0.2 -0.18571429 -0.17142857 -0.15714286 -0.14285714 -0.12857143 -0.11428571 -0.1 -0.08571429 -0.07142857 -0.05714286 -0.04285714 -0.02857143 -0.01428571 0 0 0 0 0 0
  line L17 (9.8082, 16.4039) -> (9.5546, 16.3173)
  arc A35 (8.5618, 16.7569) -> (9.5546, 16.3173) centre (9.2961, 17.0744) ccw
  arc A36 (8.5618, 16.7569) -> (8.4802, 16.94) centre (0, 13.0546) ccw
  arc A37 (8.8179, 17.9719) -> (8.4802, 16.94) centre (9.2075, 17.2732) ccw
  line L18 (8.8179, 17.9719) -> (9.0519, 18.1024)
  spline S18 degree 5 poles (9.0519, 18.1024) (9.0574, 18.1055) (9.0683, 18.1117) (9.0843, 18.1216) (9.1051, 18.1357) (9.1304, 18.1544) (9.1551, 18.1741) (9.1794, 18.1943) (9.2036, 18.2148) (9.2276, 18.2355) (9.2516, 18.2564) (9.2753, 18.2776) (9.2989, 18.2992) (9.3221, 18.3211) (9.3451, 18.3435) (9.3678, 18.3663) (9.3902, 18.3895) (9.4125, 18.4129) (9.4346, 18.4365) (9.4566, 18.4604) (9.4783, 18.4845) (9.5, 18.5088) (9.5214, 18.5334) (9.5426, 18.5583) (9.5637, 18.5834) (9.5845, 18.6088) (9.6052, 18.6344) (9.6258, 18.6602) (9.6461, 18.6862) (9.6663, 18.7124) (9.6864, 18.7389) (9.7062, 18.7655) (9.726, 18.7924) (9.7455, 18.8194) (9.7649, 18.8467) (9.7841, 18.8741) (9.8032, 18.9017) (9.8221, 18.9296) (9.8409, 18.9576) (9.8595, 18.9858) (9.8779, 19.0141) (9.8962, 19.0427) (9.9144, 19.0714) (9.9324, 19.1003) (9.9502, 19.1294) (9.9679, 19.1586) (9.9854, 19.188) (10.0028, 19.2176) (10.02, 19.2474) (10.0371, 19.2773) (10.054, 19.3073) (10.0708, 19.3375) (10.0875, 19.3679) (10.1039, 19.3985) (10.1203, 19.4291) (10.1364, 19.46) (10.1525, 19.491) (10.1684, 19.5221) (10.1841, 19.5534) (10.1997, 19.5848) (10.2151, 19.6164) (10.2304, 19.6481) (10.2455, 19.68) (10.2605, 19.712) (10.2754, 19.7441) (10.2901, 19.7764) (10.3046, 19.8088) (10.319, 19.8413) (10.3333, 19.874) (10.3474, 19.9068) (10.3614, 19.9398) (10.3724, 19.9662) (10.3806, 19.9861) (10.3861, 19.9994) (10.3888, 20.0061) knots 0 0 0 0 0 0 0.01428571 0.02857143 0.04285714 0.05714286 0.07142857 0.08571429 0.1 0.11428571 0.12857143 0.14285714 0.15714286 0.17142857 0.18571429 0.2 0.21428571 0.22857143 0.24285714 0.25714286 0.27142857 0.28571429 0.3 0.31428571 0.32857143 0.34285714 0.35714286 0.37142857 0.38571429 0.4 0.41428571 0.42857143 0.44285714 0.45714286 0.47142857 0.48571429 0.5 0.51428571 0.52857143 0.54285714 0.55714286 0.57142857 0.58571429 0.6 0.61428571 0.62857143 0.64285714 0.65714286 0.67142857 0.68571429 0.7 0.71428571 0.72857143 0.74285714 0.75714286 0.77142857 0.78571429 0.8 0.81428571 0.82857143 0.84285714 0.85714286 0.87142857 0.88571429 0.9 0.91428571 0.92857143 0.94285714 0.95714286 0.97142857 0.98571429 1 1 1 1 1 1
  arc A38 (10.3888, 20.0061) -> (9.8216, 20.7868) centre (0, 13.0546) ccw
  spline S19 degree 5 poles (9.8216, 20.7868) (9.8144, 20.7863) (9.8001, 20.7852) (9.7786, 20.7835) (9.75, 20.7812) (9.7144, 20.7781) (9.6788, 20.7748) (9.6433, 20.7714) (9.6079, 20.7677) (9.5726, 20.7639) (9.5374, 20.7599) (9.5022, 20.7557) (9.4671, 20.7514) (9.4322, 20.7468) (9.3973, 20.7421) (9.3625, 20.7371) (9.3278, 20.732) (9.2931, 20.7267) (9.2586, 20.7212) (9.2242, 20.7156) (9.1899, 20.7097) (9.1556, 20.7037) (9.1215, 20.6974) (9.0875, 20.691) (9.0536, 20.6844) (9.0197, 20.6776) (8.986, 20.6706) (8.9524, 20.6634) (8.9189, 20.656) (8.8855, 20.6484) (8.8522, 20.6406) (8.8191, 20.6326) (8.786, 20.6245) (8.7531, 20.6161) (8.7203, 20.6075) (8.6876, 20.5987) (8.6551, 20.5897) (8.6226, 20.5805) (8.5903, 20.5712) (8.5581, 20.5616) (8.5261, 20.5517) (8.4942, 20.5417) (8.4624, 20.5315) (8.4308, 20.521) (8.3993, 20.5104) (8.368, 20.4995) (8.3368, 20.4884) (8.3057, 20.477) (8.2748, 20.4655) (8.2441, 20.4537) (8.2135, 20.4417) (8.1831, 20.4294) (8.1529, 20.4169) (8.1229, 20.4041) (8.0931, 20.3911) (8.0634, 20.3779) (8.034, 20.3644) (8.0046, 20.3506) (7.9755, 20.3367) (7.9465, 20.3225) (7.9179, 20.3079) (7.8895, 20.293) (7.8614, 20.2777) (7.8336, 20.262) (7.8061, 20.2459) (7.7788, 20.2296) (7.7517, 20.2132) (7.7247, 20.1965) (7.698, 20.1796) (7.6717, 20.1622) (7.646, 20.144) (7.6262, 20.1285) (7.6119, 20.1164) (7.6025, 20.1079) (7.5979, 20.1037) knots -1 -1 -1 -1 -1 -1 -0.98571429 -0.97142857 -0.95714286 -0.94285714 -0.92857143 -0.91428571 -0.9 -0.88571429 -0.87142857 -0.85714286 -0.84285714 -0.82857143 -0.81428571 -0.8 -0.78571429 -0.77142857 -0.75714286 -0.74285714 -0.72857143 -0.71428571 -0.7 -0.68571429 -0.67142857 -0.65714286 -0.64285714 -0.62857143 -0.61428571 -0.6 -0.58571429 -0.57142857 -0.55714286 -0.54285714 -0.52857143 -0.51428571 -0.5 -0.48571429 -0.47142857 -0.45714286 -0.44285714 -0.42857143 -0.41428571 -0.4 -0.38571429 -0.37142857 -0.35714286 -0.34285714 -0.32857143 -0.31428571 -0.3 -0.28571429 -0.27142857 -0.25714286 -0.24285714 -0.22857143 -0.21428571 -0.2 -0.18571429 -0.17142857 -0.15714286 -0.14285714 -0.12857143 -0.11428571 -0.1 -0.08571429 -0.07142857 -0.05714286 -0.04285714 -0.02857143 -0.01428571 0 0 0 0 0 0
  line L19 (7.5979, 20.1037) -> (7.4015, 19.9214)
  arc A39 (6.3157, 19.9192) -> (7.4015, 19.9214) centre (6.8574, 20.5079) ccw
  arc A40 (6.3157, 19.9192) -> (6.1668, 20.0533) centre (0, 13.0546) ccw
  arc A41 (6.0555, 21.1333) -> (6.1668, 20.0533) centre (6.6957, 20.6535) ccw
  line L20 (6.0555, 21.1333) -> (6.2162, 21.3477)
  spline S20 degree 5 poles (6.2162, 21.3477) (6.22, 21.3528) (6.2274, 21.3629) (6.238, 21.3785) (6.2513, 21.3998) (6.2667, 21.4272) (6.2813, 21.4552) (6.2953, 21.4835) (6.3091, 21.5121) (6.3226, 21.5408) (6.336, 21.5697) (6.3491, 21.5987) (6.3618, 21.6279) (6.3741, 21.6575) (6.3859, 21.6873) (6.3974, 21.7173) (6.4085, 21.7476) (6.4194, 21.778) (6.4299, 21.8086) (6.4403, 21.8394) (6.4504, 21.8702) (6.4602, 21.9013) (6.4698, 21.9325) (6.4791, 21.9638) (6.4881, 21.9953) (6.4968, 22.027) (6.5053, 22.0588) (6.5136, 22.0907) (6.5216, 22.1228) (6.5294, 22.1549) (6.5369, 22.1872) (6.5443, 22.2197) (6.5514, 22.2522) (6.5582, 22.2849) (6.5649, 22.3177) (6.5713, 22.3505) (6.5774, 22.3836) (6.5834, 22.4167) (6.5891, 22.4499) (6.5947, 22.4832) (6.6, 22.5166) (6.6051, 22.5502) (6.61, 22.5838) (6.6147, 22.6175) (6.6191, 22.6513) (6.6234, 22.6852) (6.6274, 22.7192) (6.6313, 22.7533) (6.6349, 22.7875) (6.6384, 22.8218) (6.6416, 22.8561) (6.6447, 22.8905) (6.6475, 22.925) (6.6501, 22.9596) (6.6526, 22.9943) (6.6548, 23.0291) (6.6568, 23.0639) (6.6587, 23.0988) (6.6603, 23.1338) (6.6618, 23.1688) (6.6631, 23.204) (6.6641, 23.2392) (6.665, 23.2744) (6.6657, 23.3097) (6.6662, 23.3451) (6.6665, 23.3806) (6.6666, 23.4161) (6.6665, 23.4517) (6.6662, 23.4874) (6.6658, 23.5231) (6.6651, 23.5589) (6.6645, 23.5875) (6.6639, 23.609) (6.6634, 23.6234) (6.6632, 23.6306) knots 0 0 0 0 0 0 0.01428571 0.02857143 0.04285714 0.05714286 0.07142857 0.08571429 0.1 0.11428571 0.12857143 0.14285714 0.15714286 0.17142857 0.18571429 0.2 0.21428571 0.22857143 0.24285714 0.25714286 0.27142857 0.28571429 0.3 0.31428571 0.32857143 0.34285714 0.35714286 0.37142857 0.38571429 0.4 0.41428571 0.42857143 0.44285714 0.45714286 0.47142857 0.48571429 0.5 0.51428571 0.52857143 0.54285714 0.55714286 0.57142857 0.58571429 0.6 0.61428571 0.62857143 0.64285714 0.65714286 0.67142857 0.68571429 0.7 0.71428571 0.72857143 0.74285714 0.75714286 0.77142857 0.78571429 0.8 0.81428571 0.82857143 0.84285714 0.85714286 0.87142857 0.88571429 0.9 0.91428571 0.92857143 0.94285714 0.95714286 0.97142857 0.98571429 1 1 1 1 1 1
  arc A42 (6.6632, 23.6306) -> (5.8275, 24.1131) centre (0, 13.0546) ccw
  spline S21 degree 5 poles (5.8275, 24.1131) (5.8211, 24.1097) (5.8085, 24.1029) (5.7895, 24.0927) (5.7644, 24.0789) (5.7331, 24.0616) (5.7019, 24.0441) (5.6709, 24.0265) (5.6401, 24.0088) (5.6093, 23.9909) (5.5788, 23.9729) (5.5484, 23.9548) (5.5181, 23.9366) (5.488, 23.9182) (5.4581, 23.8997) (5.4283, 23.881) (5.3987, 23.8622) (5.3692, 23.8433) (5.3399, 23.8242) (5.3107, 23.8051) (5.2818, 23.7858) (5.2529, 23.7663) (5.2243, 23.7467) (5.1958, 23.727) (5.1675, 23.7072) (5.1394, 23.6872) (5.1115, 23.6671) (5.0837, 23.6468) (5.0561, 23.6265) (5.0287, 23.6059) (5.0014, 23.5853) (4.9744, 23.5645) (4.9475, 23.5436) (4.9208, 23.5226) (4.8944, 23.5014) (4.8681, 23.4801) (4.842, 23.4586) (4.8161, 23.437) (4.7904, 23.4153) (4.7649, 23.3935) (4.7396, 23.3715) (4.7145, 23.3493) (4.6897, 23.327) (4.665, 23.3046) (4.6406, 23.2821) (4.6164, 23.2594) (4.5924, 23.2365) (4.5687, 23.2136) (4.5452, 23.1905) (4.5219, 23.1672) (4.4988, 23.1438) (4.4761, 23.1202) (4.4536, 23.0965) (4.4313, 23.0726) (4.4094, 23.0486) (4.3877, 23.0244) (4.3662, 23.0001) (4.345, 22.9756) (4.3241, 22.951) (4.3034, 22.9263) (4.2831, 22.9013) (4.2633, 22.8761) (4.2438, 22.8507) (4.2249, 22.8251) (4.2063, 22.7992) (4.188, 22.7733) (4.1699, 22.7472) (4.152, 22.721) (4.1345, 22.6946) (4.1175, 22.668) (4.1015, 22.641) (4.0897, 22.6188) (4.0815, 22.6019) (4.0764, 22.5904) (4.0739, 22.5846) knots -1 -1 -1 -1 -1 -1 -0.98571429 -0.97142857 -0.95714286 -0.94285714 -0.92857143 -0.91428571 -0.9 -0.88571429 -0.87142857 -0.85714286 -0.84285714 -0.82857143 -0.81428571 -0.8 -0.78571429 -0.77142857 -0.75714286 -0.74285714 -0.72857143 -0.71428571 -0.7 -0.68571429 -0.67142857 -0.65714286 -0.64285714 -0.62857143 -0.61428571 -0.6 -0.58571429 -0.57142857 -0.55714286 -0.54285714 -0.52857143 -0.51428571 -0.5 -0.48571429 -0.47142857 -0.45714286 -0.44285714 -0.42857143 -0.41428571 -0.4 -0.38571429 -0.37142857 -0.35714286 -0.34285714 -0.32857143 -0.31428571 -0.3 -0.28571429 -0.27142857 -0.25714286 -0.24285714 -0.22857143 -0.21428571 -0.2 -0.18571429 -0.17142857 -0.15714286 -0.14285714 -0.12857143 -0.11428571 -0.1 -0.08571429 -0.07142857 -0.05714286 -0.04285714 -0.02857143 -0.01428571 0 0 0 0 0 0
  line L21 (4.0739, 22.5846) -> (3.9686, 22.3382)
  arc A43 (2.9776, 21.8945) -> (3.9686, 22.3382) centre (3.233, 22.6527) ccw
  arc A44 (2.9776, 21.8945) -> (2.787, 21.9565) centre (0, 13.0546) ccw
  arc A45 (2.2461, 22.8979) -> (2.787, 21.9565) centre (3.026, 22.7199) ccw
  line L22 (2.2461, 22.8979) -> (2.3057, 23.1591)
  spline S22 degree 5 poles (2.3057, 23.1591) (2.3071, 23.1653) (2.3097, 23.1776) (2.3131, 23.1961) (2.3166, 23.2209) (2.3195, 23.2522) (2.3214, 23.2837) (2.3227, 23.3154) (2.3236, 23.347) (2.3244, 23.3788) (2.3248, 23.4106) (2.325, 23.4424) (2.3247, 23.4743) (2.3239, 23.5063) (2.3226, 23.5383) (2.3209, 23.5705) (2.3187, 23.6026) (2.3162, 23.6348) (2.3135, 23.6671) (2.3104, 23.6994) (2.3071, 23.7317) (2.3034, 23.764) (2.2995, 23.7964) (2.2952, 23.8288) (2.2906, 23.8613) (2.2858, 23.8938) (2.2806, 23.9263) (2.2751, 23.9588) (2.2694, 23.9913) (2.2634, 24.0239) (2.2572, 24.0565) (2.2507, 24.0891) (2.244, 24.1217) (2.2369, 24.1543) (2.2297, 24.187) (2.2221, 24.2196) (2.2144, 24.2523) (2.2063, 24.285) (2.1981, 24.3177) (2.1896, 24.3504) (2.1808, 24.3831) (2.1719, 24.4158) (2.1627, 24.4485) (2.1532, 24.4812) (2.1435, 24.5139) (2.1336, 24.5466) (2.1235, 24.5793) (2.1132, 24.612) (2.1026, 24.6447) (2.0918, 24.6774) (2.0808, 24.7101) (2.0696, 24.7428) (2.0581, 24.7755) (2.0465, 24.8082) (2.0346, 24.8408) (2.0225, 24.8735) (2.0102, 24.9061) (1.9977, 24.9388) (1.985, 24.9714) (1.972, 25.004) (1.9589, 25.0366) (1.9455, 25.0692) (1.932, 25.1018) (1.9183, 25.1343) (1.9043, 25.1669) (1.8902, 25.1994) (1.8758, 25.2319) (1.8613, 25.2644) (1.8465, 25.2968) (1.8316, 25.3292) (1.8164, 25.3617) (1.8042, 25.3876) (1.7949, 25.407) (1.7886, 25.42) (1.7855, 25.4264) knots 0 0 0 0 0 0 0.01428571 0.02857143 0.04285714 0.05714286 0.07142857 0.08571429 0.1 0.11428571 0.12857143 0.14285714 0.15714286 0.17142857 0.18571429 0.2 0.21428571 0.22857143 0.24285714 0.25714286 0.27142857 0.28571429 0.3 0.31428571 0.32857143 0.34285714 0.35714286 0.37142857 0.38571429 0.4 0.41428571 0.42857143 0.44285714 0.45714286 0.47142857 0.48571429 0.5 0.51428571 0.52857143 0.54285714 0.55714286 0.57142857 0.58571429 0.6 0.61428571 0.62857143 0.64285714 0.65714286 0.67142857 0.68571429 0.7 0.71428571 0.72857143 0.74285714 0.75714286 0.77142857 0.78571429 0.8 0.81428571 0.82857143 0.84285714 0.85714286 0.87142857 0.88571429 0.9 0.91428571 0.92857143 0.94285714 0.95714286 0.97142857 0.98571429 1 1 1 1 1 1
  arc A46 (1.7855, 25.4264) -> (0.8258, 25.5273) centre (0, 13.0546) ccw
  spline S23 degree 5 poles (0.8258, 25.5273) (0.8214, 25.5216) (0.8126, 25.5103) (0.7994, 25.4932) (0.782, 25.4704) (0.7605, 25.4418) (0.7391, 25.4132) (0.718, 25.3845) (0.697, 25.3558) (0.6762, 25.327) (0.6556, 25.2981) (0.6352, 25.2692) (0.615, 25.2402) (0.5949, 25.2111) (0.5751, 25.182) (0.5555, 25.1529) (0.5361, 25.1237) (0.5168, 25.0944) (0.4978, 25.0651) (0.479, 25.0357) (0.4604, 25.0063) (0.442, 24.9768) (0.4238, 24.9473) (0.4058, 24.9177) (0.388, 24.888) (0.3704, 24.8583) (0.3531, 24.8286) (0.3359, 24.7988) (0.319, 24.769) (0.3023, 24.7391) (0.2858, 24.7091) (0.2695, 24.6792) (0.2535, 24.6491) (0.2377, 24.619) (0.2221, 24.5889) (0.2068, 24.5588) (0.1917, 24.5286) (0.1768, 24.4983) (0.1622, 24.468) (0.1478, 24.4377) (0.1336, 24.4073) (0.1197, 24.3769) (0.1061, 24.3464) (0.0927, 24.3159) (0.0795, 24.2854) (0.0667, 24.2548) (0.054, 24.2242) (0.0417, 24.1935) (0.0296, 24.1629) (0.0178, 24.1321) (0.0062, 24.1014) (-0.005, 24.0706) (-0.0159, 24.0398) (-0.0265, 24.0089) (-0.0368, 23.978) (-0.0467, 23.9471) (-0.0564, 23.9162) (-0.0659, 23.8852) (-0.075, 23.8542) (-0.0838, 23.8232) (-0.0922, 23.7921) (-0.1001, 23.7611) (-0.1075, 23.7299) (-0.1144, 23.6988) (-0.1209, 23.6676) (-0.127, 23.6364) (-0.133, 23.6052) (-0.1386, 23.574) (-0.1439, 23.5429) (-0.1486, 23.5117) (-0.1523, 23.4804) (-0.154, 23.4554) (-0.1546, 23.4366) (-0.1546, 23.424) (-0.1545, 23.4177) knots -1 -1 -1 -1 -1 -1 -0.98571429 -0.97142857 -0.95714286 -0.94285714 -0.92857143 -0.91428571 -0.9 -0.88571429 -0.87142857 -0.85714286 -0.84285714 -0.82857143 -0.81428571 -0.8 -0.78571429 -0.77142857 -0.75714286 -0.74285714 -0.72857143 -0.71428571 -0.7 -0.68571429 -0.67142857 -0.65714286 -0.64285714 -0.62857143 -0.61428571 -0.6 -0.58571429 -0.57142857 -0.55714286 -0.54285714 -0.52857143 -0.51428571 -0.5 -0.48571429 -0.47142857 -0.45714286 -0.44285714 -0.42857143 -0.41428571 -0.4 -0.38571429 -0.37142857 -0.35714286 -0.34285714 -0.32857143 -0.31428571 -0.3 -0.28571429 -0.27142857 -0.25714286 -0.24285714 -0.22857143 -0.21428571 -0.2 -0.18571429 -0.17142857 -0.15714286 -0.14285714 -0.12857143 -0.11428571 -0.1 -0.08571429 -0.07142857 -0.05714286 -0.04285714 -0.02857143 -0.01428571 0 0 0 0 0 0
  line L23 (-0.1545, 23.4177) -> (-0.1505, 23.1498)
  arc A47 (-0.8753, 22.3414) -> (-0.1505, 23.1498) centre (-0.9504, 23.1379) ccw
  arc A48 (-0.8753, 22.3414) -> (-1.0746, 22.3204) centre (0, 13.0546) ccw
  arc A49 (-1.9517, 22.9605) -> (-1.0746, 22.3204) centre (-1.1668, 23.1151) ccw
  line L24 (-1.9517, 22.9605) -> (-2.0035, 23.2234)
  spline S24 degree 5 poles (-2.0035, 23.2234) (-2.0047, 23.2295) (-2.0073, 23.2418) (-2.0118, 23.2601) (-2.0187, 23.2842) (-2.0288, 23.314) (-2.0398, 23.3436) (-2.0515, 23.373) (-2.0636, 23.4023) (-2.0758, 23.4316) (-2.0883, 23.4608) (-2.1011, 23.49) (-2.1144, 23.519) (-2.1281, 23.5479) (-2.1423, 23.5767) (-2.157, 23.6053) (-2.172, 23.6338) (-2.1874, 23.6622) (-2.203, 23.6906) (-2.219, 23.7188) (-2.2352, 23.747) (-2.2516, 23.7751) (-2.2684, 23.803) (-2.2855, 23.8309) (-2.3029, 23.8587) (-2.3205, 23.8864) (-2.3385, 23.914) (-2.3567, 23.9415) (-2.3751, 23.9689) (-2.3939, 23.9962) (-2.4128, 24.0234) (-2.432, 24.0506) (-2.4514, 24.0776) (-2.4711, 24.1046) (-2.491, 24.1314) (-2.5112, 24.1582) (-2.5316, 24.1849) (-2.5522, 24.2115) (-2.5731, 24.238) (-2.5941, 24.2644) (-2.6154, 24.2907) (-2.6369, 24.3169) (-2.6586, 24.343) (-2.6805, 24.3691) (-2.7027, 24.395) (-2.725, 24.4209) (-2.7476, 24.4467) (-2.7703, 24.4723) (-2.7933, 24.4979) (-2.8165, 24.5234) (-2.8398, 24.5488) (-2.8634, 24.5741) (-2.8871, 24.5993) (-2.9111, 24.6244) (-2.9352, 24.6494) (-2.9595, 24.6743) (-2.9841, 24.6991) (-3.0088, 24.7239) (-3.0337, 24.7485) (-3.0587, 24.773) (-3.084, 24.7975) (-3.1094, 24.8218) (-3.135, 24.846) (-3.1608, 24.8702) (-3.1868, 24.8942) (-3.213, 24.9182) (-3.2393, 24.9421) (-3.2658, 24.9658) (-3.2925, 24.9895) (-3.3193, 25.013) (-3.3463, 25.0365) (-3.3681, 25.0552) (-3.3845, 25.0691) (-3.3954, 25.0784) (-3.4009, 25.0831) knots 0 0 0 0 0 0 0.01428571 0.02857143 0.04285714 0.05714286 0.07142857 0.08571429 0.1 0.11428571 0.12857143 0.14285714 0.15714286 0.17142857 0.18571429 0.2 0.21428571 0.22857143 0.24285714 0.25714286 0.27142857 0.28571429 0.3 0.31428571 0.32857143 0.34285714 0.35714286 0.37142857 0.38571429 0.4 0.41428571 0.42857143 0.44285714 0.45714286 0.47142857 0.48571429 0.5 0.51428571 0.52857143 0.54285714 0.55714286 0.57142857 0.58571429 0.6 0.61428571 0.62857143 0.64285714 0.65714286 0.67142857 0.68571429 0.7 0.71428571 0.72857143 0.74285714 0.75714286 0.77142857 0.78571429 0.8 0.81428571 0.82857143 0.84285714 0.85714286 0.87142857 0.88571429 0.9 0.91428571 0.92857143 0.94285714 0.95714286 0.97142857 0.98571429 1 1 1 1 1 1
  arc A50 (-3.4009, 25.0831) -> (-4.3187, 24.7848) centre (0, 13.0546) ccw
  spline S25 degree 5 poles (-4.3187, 24.7848) (-4.3205, 24.7779) (-4.3239, 24.7639) (-4.3289, 24.743) (-4.3355, 24.7151) (-4.3436, 24.6802) (-4.3515, 24.6454) (-4.3591, 24.6106) (-4.3666, 24.5758) (-4.3739, 24.541) (-4.381, 24.5062) (-4.3879, 24.4715) (-4.3945, 24.4368) (-4.401, 24.4021) (-4.4073, 24.3675) (-4.4133, 24.3329) (-4.4192, 24.2983) (-4.4249, 24.2637) (-4.4303, 24.2292) (-4.4356, 24.1947) (-4.4406, 24.1603) (-4.4454, 24.1258) (-4.45, 24.0914) (-4.4544, 24.0571) (-4.4586, 24.0228) (-4.4626, 23.9885) (-4.4664, 23.9543) (-4.4699, 23.9201) (-4.4732, 23.886) (-4.4763, 23.8519) (-4.4792, 23.8178) (-4.4819, 23.7838) (-4.4843, 23.7498) (-4.4865, 23.7159) (-4.4885, 23.6821) (-4.4903, 23.6483) (-4.4918, 23.6145) (-4.4931, 23.5808) (-4.4941, 23.5472) (-4.4949, 23.5136) (-4.4955, 23.4801) (-4.4958, 23.4467) (-4.4959, 23.4133) (-4.4957, 23.38) (-4.4953, 23.3468) (-4.4946, 23.3136) (-4.4937, 23.2805) (-4.4925, 23.2475) (-4.4911, 23.2145) (-4.4894, 23.1817) (-4.4874, 23.1489) (-4.4852, 23.1162) (-4.4826, 23.0836) (-4.4797, 23.0511) (-4.4765, 23.0187) (-4.4731, 22.9864) (-4.4694, 22.9542) (-4.4654, 22.9221) (-4.4611, 22.89) (-4.4565, 22.8581) (-4.4516, 22.8263) (-4.4461, 22.7947) (-4.4403, 22.7633) (-4.4339, 22.732) (-4.4271, 22.7009) (-4.4201, 22.6699) (-4.4128, 22.639) (-4.4053, 22.6082) (-4.3974, 22.5776) (-4.389, 22.5471) (-4.3796, 22.5171) (-4.3711, 22.4935) (-4.3639, 22.4761) (-4.3588, 22.4647) (-4.3562, 22.4589) knots -1 -1 -1 -1 -1 -1 -0.98571429 -0.97142857 -0.95714286 -0.94285714 -0.92857143 -0.91428571 -0.9 -0.88571429 -0.87142857 -0.85714286 -0.84285714 -0.82857143 -0.81428571 -0.8 -0.78571429 -0.77142857 -0.75714286 -0.74285714 -0.72857143 -0.71428571 -0.7 -0.68571429 -0.67142857 -0.65714286 -0.64285714 -0.62857143 -0.61428571 -0.6 -0.58571429 -0.57142857 -0.55714286 -0.54285714 -0.52857143 -0.51428571 -0.5 -0.48571429 -0.47142857 -0.45714286 -0.44285714 -0.42857143 -0.41428571 -0.4 -0.38571429 -0.37142857 -0.35714286 -0.34285714 -0.32857143 -0.31428571 -0.3 -0.28571429 -0.27142857 -0.25714286 -0.24285714 -0.22857143 -0.21428571 -0.2 -0.18571429 -0.17142857 -0.15714286 -0.14285714 -0.12857143 -0.11428571 -0.1 -0.08571429 -0.07142857 -0.05714286 -0.04285714 -0.02857143 -0.01428571 0 0 0 0 0 0
  line L25 (-4.3562, 22.4589) -> (-4.2435, 22.2158)
  arc A51 (-4.5769, 21.1825) -> (-4.2435, 22.2158) centre (-4.9694, 21.8796) ccw
  arc A52 (-4.5769, 21.1825) -> (-4.7505, 21.0823) centre (0, 13.0546) ccw
  arc A53 (-5.8121, 21.3102) -> (-4.7505, 21.0823) centre (-5.1579, 21.7708) ccw
  line L26 (-5.8121, 21.3102) -> (-5.9663, 21.5293)
  spline S26 degree 5 poles (-5.9663, 21.5293) (-5.9699, 21.5345) (-5.9773, 21.5446) (-5.9888, 21.5595) (-6.005, 21.5788) (-6.0263, 21.6019) (-6.0484, 21.6244) (-6.071, 21.6465) (-6.0939, 21.6684) (-6.1171, 21.6902) (-6.1404, 21.7118) (-6.1639, 21.7332) (-6.1878, 21.7543) (-6.2121, 21.7751) (-6.2368, 21.7956) (-6.2618, 21.8158) (-6.2872, 21.8358) (-6.3128, 21.8555) (-6.3386, 21.875) (-6.3646, 21.8943) (-6.3909, 21.9134) (-6.4174, 21.9324) (-6.4441, 21.9511) (-6.471, 21.9697) (-6.4982, 21.988) (-6.5256, 22.0061) (-6.5532, 22.024) (-6.581, 22.0417) (-6.609, 22.0592) (-6.6372, 22.0766) (-6.6656, 22.0937) (-6.6942, 22.1107) (-6.723, 22.1275) (-6.7519, 22.1442) (-6.781, 22.1606) (-6.8103, 22.1768) (-6.8398, 22.1929) (-6.8695, 22.2088) (-6.8993, 22.2246) (-6.9293, 22.2401) (-6.9594, 22.2555) (-6.9897, 22.2707) (-7.0202, 22.2858) (-7.0508, 22.3006) (-7.0816, 22.3153) (-7.1125, 22.3299) (-7.1436, 22.3442) (-7.1748, 22.3584) (-7.2062, 22.3724) (-7.2377, 22.3863) (-7.2694, 22.4) (-7.3012, 22.4135) (-7.3332, 22.4269) (-7.3652, 22.4401) (-7.3975, 22.4531) (-7.4298, 22.466) (-7.4623, 22.4787) (-7.495, 22.4912) (-7.5277, 22.5036) (-7.5606, 22.5158) (-7.5936, 22.5279) (-7.6267, 22.5398) (-7.66, 22.5515) (-7.6934, 22.5631) (-7.7269, 22.5745) (-7.7606, 22.5857) (-7.7943, 22.5968) (-7.8282, 22.6077) (-7.8622, 22.6185) (-7.8963, 22.6291) (-7.9305, 22.6395) (-7.958, 22.6477) (-7.9786, 22.6538) (-7.9924, 22.6579) (-7.9993, 22.6599) knots 0 0 0 0 0 0 0.01428571 0.02857143 0.04285714 0.05714286 0.07142857 0.08571429 0.1 0.11428571 0.12857143 0.14285714 0.15714286 0.17142857 0.18571429 0.2 0.21428571 0.22857143 0.24285714 0.25714286 0.27142857 0.28571429 0.3 0.31428571 0.32857143 0.34285714 0.35714286 0.37142857 0.38571429 0.4 0.41428571 0.42857143 0.44285714 0.45714286 0.47142857 0.48571429 0.5 0.51428571 0.52857143 0.54285714 0.55714286 0.57142857 0.58571429 0.6 0.61428571 0.62857143 0.64285714 0.65714286 0.67142857 0.68571429 0.7 0.71428571 0.72857143 0.74285714 0.75714286 0.77142857 0.78571429 0.8 0.81428571 0.82857143 0.84285714 0.85714286 0.87142857 0.88571429 0.9 0.91428571 0.92857143 0.94285714 0.95714286 0.97142857 0.98571429 1 1 1 1 1 1
  arc A54 (-7.9993, 22.6599) -> (-8.7165, 22.0141) centre (0, 13.0546) ccw
  spline S27 degree 5 poles (-8.7165, 22.0141) (-8.7152, 22.0071) (-8.7126, 21.9929) (-8.7087, 21.9717) (-8.7034, 21.9436) (-8.6966, 21.9084) (-8.6896, 21.8734) (-8.6825, 21.8385) (-8.6752, 21.8036) (-8.6677, 21.7689) (-8.66, 21.7343) (-8.6522, 21.6998) (-8.6442, 21.6654) (-8.636, 21.631) (-8.6276, 21.5968) (-8.6191, 21.5628) (-8.6104, 21.5288) (-8.6015, 21.4949) (-8.5924, 21.4611) (-8.5832, 21.4275) (-8.5738, 21.394) (-8.5642, 21.3606) (-8.5544, 21.3273) (-8.5445, 21.2941) (-8.5343, 21.261) (-8.524, 21.2281) (-8.5135, 21.1953) (-8.5029, 21.1626) (-8.492, 21.1301) (-8.481, 21.0977) (-8.4698, 21.0654) (-8.4584, 21.0333) (-8.4468, 21.0013) (-8.435, 20.9694) (-8.423, 20.9376) (-8.4109, 20.9061) (-8.3985, 20.8746) (-8.386, 20.8433) (-8.3733, 20.8122) (-8.3604, 20.7812) (-8.3473, 20.7503) (-8.334, 20.7196) (-8.3205, 20.6891) (-8.3068, 20.6588) (-8.2929, 20.6286) (-8.2788, 20.5985) (-8.2645, 20.5687) (-8.2499, 20.539) (-8.2352, 20.5095) (-8.2203, 20.4801) (-8.2052, 20.451) (-8.1898, 20.422) (-8.1742, 20.3933) (-8.1584, 20.3648) (-8.1423, 20.3365) (-8.126, 20.3084) (-8.1095, 20.2805) (-8.0928, 20.2527) (-8.0759, 20.2252) (-8.0587, 20.1979) (-8.0412, 20.1709) (-8.0234, 20.1442) (-8.0053, 20.1179) (-7.9867, 20.0919) (-7.9679, 20.0663) (-7.9488, 20.0408) (-7.9296, 20.0156) (-7.9102, 19.9905) (-7.8906, 19.9657) (-7.8705, 19.9413) (-7.8498, 19.9177) (-7.8323, 19.8996) (-7.8187, 19.8866) (-7.8094, 19.8782) (-7.8046, 19.8741) knots -1 -1 -1 -1 -1 -1 -0.98571429 -0.97142857 -0.95714286 -0.94285714 -0.92857143 -0.91428571 -0.9 -0.88571429 -0.87142857 -0.85714286 -0.84285714 -0.82857143 -0.81428571 -0.8 -0.78571429 -0.77142857 -0.75714286 -0.74285714 -0.72857143 -0.71428571 -0.7 -0.68571429 -0.67142857 -0.65714286 -0.64285714 -0.62857143 -0.61428571 -0.6 -0.58571429 -0.57142857 -0.55714286 -0.54285714 -0.52857143 -0.51428571 -0.5 -0.48571429 -0.47142857 -0.45714286 -0.44285714 -0.42857143 -0.41428571 -0.4 -0.38571429 -0.37142857 -0.35714286 -0.34285714 -0.32857143 -0.31428571 -0.3 -0.28571429 -0.27142857 -0.25714286 -0.24285714 -0.22857143 -0.21428571 -0.2 -0.18571429 -0.17142857 -0.15714286 -0.14285714 -0.12857143 -0.11428571 -0.1 -0.08571429 -0.07142857 -0.05714286 -0.04285714 -0.02857143 -0.01428571 0 0 0 0 0 0
  line L27 (-7.8046, 19.8741) -> (-7.6029, 19.6978)
  arc A55 (-7.4871, 18.6182) -> (-7.6029, 19.6978) centre (-8.1292, 19.0953) ccw
  arc A56 (-7.4871, 18.6182) -> (-7.6049, 18.456) centre (0, 13.0546) ccw
  arc A57 (-8.6674, 18.2325) -> (-7.6049, 18.456) centre (-8.2572, 18.9193) ccw
  line L28 (-8.6674, 18.2325) -> (-8.8975, 18.3699)